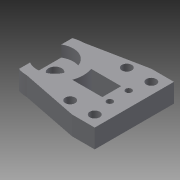
# Autodesk Inventor part: servo_clip_holder2_final
Saved by Autodesk Inventor 2015 (Build 190159000, 159)
## iProperties
Created: 2017-12-03
Part Number: servo_clip_holder2_final
Material: Generic
Document SubType Name: Modeling
Designer: Anshul
Density: 1 g/cm^3
Appearance: Default
Author: Anshul
Autodesk Inventor part; units mm, degrees
ref_plane "YZ Plane" through (0, 0, 0) normal (1, 0, 0) x (0, 1, 0)
ref_plane "XZ Plane" through (0, 0, 0) normal (0, 1, 0) x (-1, 0, 0)
ref_plane "XY Plane" through (0, 0, 0) normal (0, 0, 1) x (1, 0, 0)
sketch "Sketch1" plane through (0, 0, 0) normal (0, 1, 0) x (-1, 0, 0)
  line L0 (0, 0) -> (0, -42)
  line L1 (0, -42) -> (12, -42)
  line L2 (12, -42) -> (12, 0)
  line L3 (12, 0) -> (0, 0)
  line L4 (0, -21) -> (0, -26)
  line L5 (0, -21) -> (0, -16)
  line L6 (0, -16) -> (0, -19)
  line L7 (0, -16) -> (0, -13)
  line L8 (0, -26) -> (0, -23)
  line L9 (0, -26) -> (0, -29)
  line L10 (0, -29) -> (12, -29)
  line L11 (0, -13) -> (12, -13)
  line L12 (6.4, -16) -> (12, -16)
  line L13 (6.4, -26) -> (12, -26)
  line L14 (12, -16) -> (8, -16)
  circle A0 centre (8, -16) radius 1.6
  circle A1 centre (8, -26) radius 1.6
  line L15 (12, -26) -> (8, -26)
  dimension "d9" = 3.2
  dimension "d10" = 3.2
  dimension "d0" = 42
  dimension "d1" = 12
  dimension "d2" = 5
  dimension "d3" = 5
  dimension "d4" = 3
  dimension "d5" = 3
  dimension "d6" = 3
  dimension "d7" = 3
  dimension "d8" = 4
  constraints: 32 end point, 12 point on line, 6 perpendicular, 2 horizontal alignment, 1 coincident, 1 horizontal, 1 midpoint, 1 parallel, 1 vertical, 4 other
  measures "d0" distance of L0.start L0.end
  measures "d1" distance of L0.end L1.end
  measures "d2" distance of L4.start L4.end
  measures "d3" distance of L4.start L5.end
  measures "d4" distance of L5.end L6.end
  measures "d5" distance of L5.end L7.end
  measures "d6" distance of L4.end L8.end
  measures "d7" distance of L4.end L9.end
  measures "d8" distance of L12.end L14.end
extrude "Extrusion1" add sketch "Sketch1" along normal blind 15
sketch "Sketch2" plane through (0, 0, 0) normal (0, -1, 0) x (1, 0, 0)
  line L0 (-12, 0) -> (-12, -42)
  line L1 (-12, -42) -> (-12, 0) projected
  line L2 (-12, -21) -> (-42, -21)
  circle A0 centre (-42, -21) radius 3.5
  arc A1 (-47, -35.1421) -> (-47, -6.8579) centre (-42, -21) ccw
  line L3 (-42, -21) -> (-47, -21)
  line L4 (-47, -21) -> (-47, -35.1421)
  line L5 (-47, -21) -> (-47, -6.8579)
  line L6 (-42, -36) -> (-12, -42)
  line L7 (-42, -6) -> (-12, 0)
  line L8 (-12, -42) -> (0, -42)
  line L9 (0, -42) -> (0, 0)
  line L10 (0, 0) -> (0, -42) projected
  line L11 (0, 0) -> (-12, 0)
  circle A2 centre (-8, -16) radius 1.6 projected
  circle A3 centre (-8, -16) radius 1.6
  circle A4 centre (-8, -26) radius 1.6 projected
  circle A5 centre (-8, -26) radius 1.6
  line L12 (-12, -42) -> (-12, -36.5)
  line L13 (-12, 0) -> (-12, -5.5)
  line L14 (-17, -6.5) -> (-32.2985, -9.5597)
  line L15 (-32.2985, -32.4403) -> (-17, -35.5)
  circle A6 centre (-42, -21) radius 5
  line L16 (-12, -21) -> (-17, -21)
  line L17 (-17, -16) -> (-17, -6.5)
  line L18 (-17, -26) -> (-17, -35.5)
  line L19 (-42, -16) -> (-33.9223, -16)
  line L20 (-27.8579, -16) -> (-12, -16)
  line L21 (-42, -26) -> (-33.9223, -26)
  line L22 (-27.8579, -26) -> (-12, -26)
  arc A7 (-47, -29.2536) -> (-47, -12.7464) centre (-42, -21) ccw
  line L23 (-12, -21) -> (-12, -31)
  line L24 (-12, -31) -> (-25, -31)
  line L25 (-25, -31) -> (-25, -41)
  line L26 (-25, -41) -> (0, -41)
  line L27 (-12, -21) -> (-12, -11)
  line L28 (-12, -11) -> (-25, -11)
  line L29 (-25, -11) -> (-25, -1)
  line L30 (-25, -1) -> (0, -1)
  line L31 (0, -1) -> (0, -6)
  line L32 (0, -6) -> (-6, -6)
  line L33 (-25, -1) -> (-25, -6)
  line L34 (-25, -6) -> (-19, -6)
  line L35 (-25, -31) -> (-25, -36)
  line L36 (-25, -36) -> (-19, -36)
  circle A8 centre (-19, -36) radius 2.6
  line L37 (0, -41) -> (0, -36)
  line L38 (0, -36) -> (-6, -36)
  circle A9 centre (-6, -36) radius 2.6
  circle A10 centre (-6, -6) radius 2.6
  circle A11 centre (-19, -6) radius 2.6
  line L39 (-27.8579, -16) -> (-12, -16)
  line L40 (-12, -16) -> (-12, -26)
  line L41 (-12, -26) -> (-27.8579, -26)
  point P0 (-47, -12.9223)
  point P1 (-47, -29.0777)
  dimension "d13" = 30
  dimension "d14" = 7
  dimension "d16" = 30
  dimension "d17" = 5
  dimension "d30" = 5.5
  dimension "d31" = 5.5
  dimension "d32" = 10
  dimension "d33" = 5
  dimension "d36" = 19.3
  dimension "d39" = 10
  dimension "d40" = 13
  dimension "d41" = 10
  dimension "d42" = 25
  dimension "d48" = 10
  dimension "d49" = 13
  dimension "d50" = 10
  dimension "d51" = 25
  dimension "d52" = 5
  dimension "d53" = 6
  dimension "d54" = 6
  dimension "d55" = 5
  dimension "d56" = 6
  dimension "d57" = 5.2
  dimension "d58" = 5
  dimension "d59" = 6
  dimension "d60" = 5.2
  dimension "d61" = 5.2
  dimension "d62" = 5.2
  constraints: 80 end point, 20 point on line, 12 perpendicular, 12 point on circle, 10 centre point, 9 coincident, 5 collinear, 4 parallel, 4 tangent, 3 horizontal, 3 midpoint
  measures "d13" distance of L2.start L2.end
  measures "d14" diameter of A0
  measures "d16" diameter of A1
  measures "d17" distance of L3.start L3.end
  measures "d30" distance of L0.end L12.end
  measures "d31" distance of L0.start L13.end
  measures "d32" diameter of A6
  measures "d33" distance of L2.start L16.end
  measures "d36" diameter of A7
  measures "d39" distance of L2.start L23.end
  measures "d40" distance of L23.end L24.end
  measures "d41" distance of L24.end L25.end
  measures "d42" distance of L25.end L26.end
  measures "d48" distance of L2.start L27.end
  measures "d49" distance of L27.end L28.end
  measures "d50" distance of L28.end L29.end
  measures "d51" distance of L29.end L30.end
  measures "d52" distance of L30.end L31.end
  measures "d53" distance of L31.end L32.end
  measures "d54" distance of L33.end L34.end
  measures "d55" distance of L24.end L35.end
  measures "d56" distance of L35.end L36.end
  measures "d57" diameter of A8
  measures "d58" distance of L26.end L37.end
  measures "d59" distance of L37.end L38.end
  measures "d60" diameter of A9
  measures "d61" diameter of A10
  measures "d62" diameter of A11
extrude "Extrusion2" add sketch "Sketch2" along normal blind 10 contours A9 | A10 | L0 L30 L9 L26 | L0 L28 L17 A11 L34 L29 L7 L30 | L0 L20 L17 L28 | L30 L7 L0 | L0 L11 L9 L30 | L0 L2 A1 L20 | L28 L29 L14 A11 L17 | L17 L20 A1 L14 L29 L28 | L0 L22 A1 L2 | A11 L14 L17 | L17 L14 A11 | L29 L14 A1 L7 | L0 L24 L18 L22 | A1 L2 A7 L5 | L14 L29 L34 A11 | L0 L26 L6 L25 L36 A8 L18 L24 | L18 L24 L25 L15 A1 L22 | A1 L4 A7 L2 | L9 L8 L0 L26 | L18 A8 L15 L25 L24 | A7 L4 A6 L2 | L2 A6 L5 A7 | L0 L6 L26 | A8 L15 L18 | L18 L15 A8 | L15 L25 L6 A1 | A6 L3 A0 L2 | L2 A0 L3 A6 | A8 L36 L25 L15
extrude "Extrusion6" cut sketch "Sketch2" along normal blind 6 contours A7 L4 A6 L2 | L2 A6 L5 A7 | A6 L3 A0 L2 | L2 A0 L3 A6
extrude "Extrusion7" cut sketch "Sketch2" along normal mid plane 40 contours A9 | A10 | L0 L2 A1 L20 | L0 L22 A1 L2 | A11 L14 L17 | L17 L14 A11 | A8 L15 L18 | L18 L15 A8
extrude "Extrusion8" cut sketch "Sketch2" against normal blind 40 contours A9 | A10 | L0 L30 L9 L26 | L0 L28 L17 A11 L34 L29 L7 L30 | L0 L11 L9 L30 | L28 L29 L14 A11 L17 | L7 L29 L30 | L14 L29 L34 A11 | L0 L26 L6 L25 L36 A8 L18 L24 | L9 L8 L0 L26 | L18 A8 L15 L25 L24 | L26 L25 L6 | A8 L36 L25 L15 | A2 | A4
body "Solid1"
